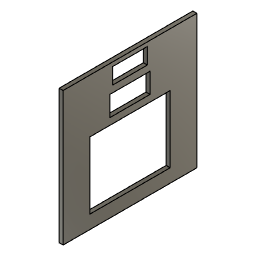
Grid Power Fascia v1 (Autodesk Fusion 360 design; units mm, degrees)
Autodesk Fusion 360 part; units mm, degrees
sketch "Sketch1" plane through (0, 0, 0) normal (1, 0, 0) x (0, 1, 0)
  line L0 (0, 0) -> (100, 0)
  line L1 (100, 0) -> (100, 100)
  line L2 (100, 100) -> (0, 100)
  line L3 (0, 100) -> (0, 0)
  line L4 (50, 10) -> (80, 10)
  line L5 (50, 60) -> (20, 60)
  line L6 (20, 60) -> (80, 60)
  line L7 (80, 60) -> (80, 10)
  line L8 (80, 10) -> (20, 10)
  line L9 (20, 10) -> (20, 60)
  line L10 (35, 65) -> (65, 65)
  line L11 (65, 65) -> (65, 80)
  line L12 (65, 80) -> (35, 80)
  line L13 (35, 80) -> (35, 65)
  line L14 (50, 85) -> (63, 85)
  line L15 (50, 97) -> (37, 97)
  line L16 (37, 97) -> (63, 97)
  line L17 (63, 97) -> (63, 85)
  line L18 (63, 85) -> (37, 85)
  line L19 (37, 85) -> (37, 97)
  dimension "d1" = 100
  dimension "d2" = 100
  dimension "d4" = 30
  dimension "d5" = 13
  dimension "d6" = 12
  dimension "d7" = 13
  constraint horizontal L0
  constraint vertical L1
  constraint horizontal L2
  constraint vertical L3
  constraint coincident L0.start L3.end
  constraint horizontal L6
  constraint vertical L7
  constraint horizontal L8
  constraint vertical L9
  constraint horizontal L10
  constraint vertical L11
  constraint horizontal L12
  constraint vertical L13
  constraint horizontal L14
  constraint horizontal L16
  constraint vertical L17
  constraint horizontal L18
  constraint vertical L19
  measures "d1" distance of L0.start L0.end
  measures "d2" distance of L0.start L2.end
  measures "d4" distance of L4.start L4.end
  measures "d5" distance of L14.start L14.end
  measures "d6" distance of L14.start L15.start
  measures "d7" distance of L15.start L15.end
extrude "Extrude1" add sketch "Sketch1" along normal blind 3
